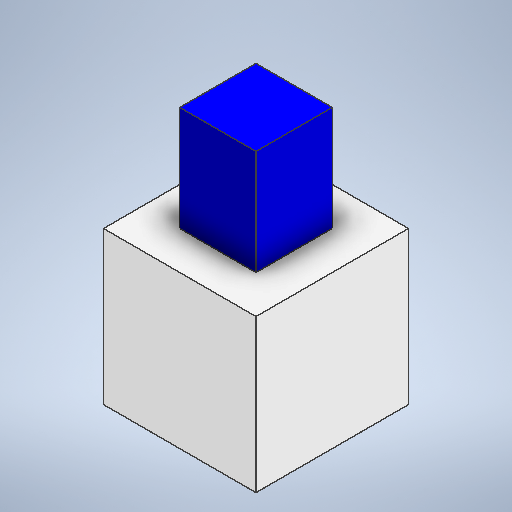
# Autodesk Inventor part: switch
Saved by Autodesk Inventor 2025 (Build 290162000, 162)
## iProperties
Created: 2026-02-25
Part Number: switch
Material: 一般
Document SubType Name: Modeling
Designer: sooo1
Density: 1 g/cm^3
Appearance: 既定
Author: sooo1
Autodesk Inventor part; units mm, degrees
ref_plane "YZ Plane" through (0, 0, 0) normal (1, 0, 0) x (0, 1, 0)
ref_plane "XZ Plane" through (0, 0, 0) normal (0, 1, 0) x (-1, 0, 0)
ref_plane "XY Plane" through (0, 0, 0) normal (0, 0, 1) x (1, 0, 0)
sketch "スケッチ1" plane through (0, 0, 0) normal (0, 1, 0) x (-1, 0, 0)
  line L0 (4, 4) -> (-4, 4)
  line L1 (-4, 4) -> (-4, -4)
  line L2 (-4, -4) -> (4, -4)
  line L3 (4, -4) -> (4, 4)
  line L4 (4, 4) -> (-4, -4) construction
  line L5 (-4, 4) -> (4, -4) construction
  point P0 (0, 0)
  dimension "d0" = 8
  constraints: 12 end point, 2 midpoint, 2 parallel, 2 perpendicular, 1 horizontal
  measures "d0" distance of L2.end L0.start
extrude "押し出し1" add sketch "スケッチ1" along normal blind 8
sketch "スケッチ2" plane through (0, 8, 0) normal (0, 1, 0) x (1, 0, 0)
  line L0 (-2, -2) -> (2, -2)
  line L1 (2, -2) -> (2, 2)
  line L2 (2, 2) -> (-2, 2)
  line L3 (-2, 2) -> (-2, -2)
  line L4 (-2, -2) -> (2, 2) construction
  line L5 (2, -2) -> (-2, 2) construction
  point P0 (0, 0)
  dimension "d4" = 4
  constraints: 12 end point, 2 midpoint, 2 parallel, 2 perpendicular, 1 horizontal
  measures "d4" distance of L2.end L0.start
extrude "押し出し2" add sketch "スケッチ2" along normal blind 5.5
